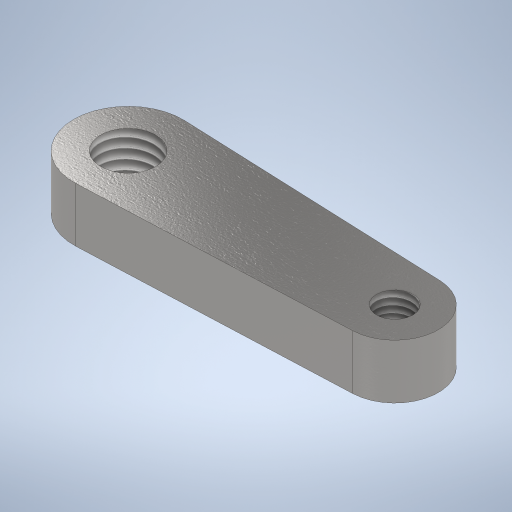
# Autodesk Inventor part: Kurbelarm
Saved by Autodesk Inventor 2024 (Build 280153000, 153)
## iProperties
Created: 2024-03-01
Part Number: Kurbelarm
Material: Stahl, galvanisiert
Document SubType Name: Modeling
Designer: ffogue
Density: 7.85 g/cm^3
Appearance: Galvanisiert
Author: ffogue
Autodesk Inventor part; units mm, degrees
ref_plane "YZ Plane" through (0, 0, 0) normal (1, 0, 0) x (0, 1, 0)
ref_plane "XZ Plane" through (0, 0, 0) normal (0, 1, 0) x (-1, 0, 0)
ref_plane "XY Plane" through (0, 0, 0) normal (0, 0, 1) x (1, 0, 0)
sketch "Skizze1" plane through (0, 0, 0) normal (0, 0, 1) x (1, 0, 0)
  arc A0 (10.4173, 10) -> (10.4173, -10) centre (10.0084, 0) ccw
  line L0 (10.4173, 10) -> (59.3205, 8)
  line L1 (10.4173, -10) -> (59.3205, -8)
  arc A1 (59.3205, -8) -> (59.3205, 8) centre (58.9933, 0) ccw
  point P0 (0, 0)
  point P1 (67, 0)
  point P2 (0, 0)
  dimension "d0" = 20
  dimension "d1" = 16
  dimension "d2" = 67
  constraints: 6 point on circle, 4 end point, 4 tangent, 2 centre point, 1 coincident, 1 horizontal alignment, 1 vertical alignment
  measures "d0" distance of L1.start L0.start
  measures "d1" distance of L1.end L0.end
  measures "d2" distance of point (67, 0) point (0, 0)
extrude "Extrusion1" add sketch "Skizze1" along normal blind 10
sketch "Skizze2" plane through (0, 0, 10) normal (0, 0, 1) x (1, 0, 0)
  arc A0 (10.4173, 10) -> (10.4173, -10) centre (10.0084, 0) ccw projected
  point P0 (0, 0)
  constraints: 1 coincident
hole "Bohrung1" at (10.0084, 0, 10) direction (0, 0, -1) diameter 10.106 end through all thread size "M12x1.75" class "6H" standard "ISO Metric profile"
sketch "Skizze3" plane through (0, 0, 10) normal (0, 0, 1) x (1, 0, 0)
  arc A0 (59.3205, -8) -> (59.3205, 8) centre (58.9933, 0) ccw projected
  point P0 (0, 0)
  constraints: 1 coincident
hole "Bohrung2" at (58.9933, 0, 10) direction (0, 0, -1) diameter 6.647 end through all thread size "M8x1.25" class "6H" standard "ISO Metric profile"
